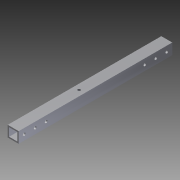
# Autodesk Inventor part: towermiddleunderthing
Saved by Autodesk Inventor 2011 SP1 (Build 150282100, 282)
## iProperties
Created: 2012-01-18
Part Number: towermiddleunderthing
Document SubType Name: Modeling
Designer: Christopher
Density: 1 g/cm^3
Author: Christopher
Autodesk Inventor part; units mm, degrees
ref_plane "YZ Plane" through (0, 0, 0) normal (1, 0, 0) x (0, 1, 0)
ref_plane "XZ Plane" through (0, 0, 0) normal (0, 1, 0) x (-1, 0, 0)
ref_plane "XY Plane" through (0, 0, 0) normal (0, 0, 1) x (1, 0, 0)
sketch "Sketch1" plane through (0, 0, 0) normal (0, 0, 1) x (1, 0, 0)
  line L0 (0, 0) -> (25.4, 0)
  line L1 (25.4, 0) -> (25.4, 25.4)
  line L2 (25.4, 25.4) -> (0, 25.4)
  line L3 (0, 25.4) -> (0, 0)
  line L4 (3.175, 22.225) -> (22.225, 22.225)
  line L5 (22.225, 22.225) -> (22.225, 3.175)
  line L6 (22.225, 3.175) -> (3.175, 3.175)
  line L7 (3.175, 3.175) -> (3.175, 22.225)
  dimension "d0" = 25.4
  dimension "d1" = 25.4
  dimension "d2" = 3.175
  constraints: 16 end point, 4 parallel, 2 perpendicular, 1 horizontal, 3 other
  measures "d0" distance of L1.end L2.end
  measures "d1" distance of L0.end L1.end
  measures "d2" distance between parallel lines of L3 L7
extrude "Extrusion1" add sketch "Sketch1" against normal blind 355.6
sketch "Sketch2" plane through (0, 0, 0) normal (-1, 0, 0) x (0, 0, 1)
  line L0 (0, 25.4) -> (-355.6, 25.4) projected
  line L1 (0, 25.4) -> (0, 0) projected
  point P0 (-317.5, 12.7)
  point P1 (-292.1, 12.7)
  point P2 (-12.7, 12.7)
  point P3 (-38.1, 12.7)
  point P4 (-63.5, 12.7)
  point P5 (-317.5, 12.7)
  point P6 (-342.9, 12.7)
  dimension "d6" = 25.4
  dimension "d7" = 12.7
  dimension "d24" = 12.7
  dimension "d25" = 25.4
  dimension "d26" = 25.4
  dimension "d27" = 25.4
  dimension "d31" = 25.4
  dimension "d32" = 228.6
  measures "d6" distance of point (-292.1, 12.7) point (-317.5, 12.7)
  measures "d7" distance from line of L0 point (-317.5, 12.7)
  measures "d24" distance from line of L1 point (-12.7, 12.7)
  measures "d25" distance of point (-12.7, 12.7) point (-38.1, 12.7)
  measures "d26" distance of point (-292.1, 12.7) point (-317.5, 12.7)
  measures "d27" distance of point (-38.1, 12.7) point (-63.5, 12.7)
  measures "d31" distance of point (-342.9, 12.7) point (-317.5, 12.7)
  measures "d32" distance of point (-292.1, 12.7) point (-63.5, 12.7)
hole "Hole1" at (0, 12.7, -317.5) at (0, 12.7, -292.1) at (0, 12.7, -38.1) at (0, 12.7, -12.7) at (0, 12.7, -63.5) at (0, 12.7, -342.9) direction (1, 0, 0) diameter 6.35 depth 25.4 tip angle 118
sketch "Sketch5" plane through (0, 25.4, 0) normal (0, 1, 0) x (1, 0, 0)
  line L0 (25.4, 0) -> (0, 0) projected
  point P0 (12.7, 152.4)
  dimension "d34" = 152.4
  measures "d34" distance from line of point (12.7, 152.4) L0
hole "Hole3" at (12.7, 25.4, -152.4) direction (0, -1, 0) diameter 6.35 depth 25.4 tip angle 118
body "Solid1"
